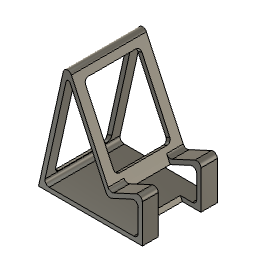
MultimeterStand (Autodesk Fusion 360 design; units mm, degrees)
Autodesk Fusion 360 part; units mm, degrees
sketch "Sketch11" plane through (0, 0, 0) normal (0, 1, 0) x (1, 0, 0)
  line L0 (0, 0) -> (0, -35) construction
  line L1 (0, -35) -> (38.0649, -52.75)
  line L2 (0, -35) -> (42, -35) construction
  line L3 (38.0649, -52.75) -> (38.0649, 0)
  line L4 (0, -35) -> (-48.0728, -138.0925)
  line L5 (0, -35) -> (131.25, -35) construction
  line L6 (-48.0728, -138.0925) -> (-53.0728, -138.0925)
  line L7 (0, 0) -> (61, 0) construction
  line L8 (-53.0728, -138.0925) -> (-83.6872, 0)
  line L9 (-53.0728, -138.0925) -> (72.8842, -138.0925) construction
  line L10 (0, 0) -> (-120, 0) construction
  line L11 (-83.6872, 0) -> (38.0649, 0)
  dimension "d68" = 35
  dimension "d69" = 42
  dimension "d70" = 25
  dimension "d71" = 115
  dimension "d72" = 113.75
  dimension "d73" = 5
  dimension "d81" = 102.5
  constraint vertical L0
  constraint coincident L0.start L7.start
  constraint horizontal L2
  constraint vertical L3
  constraint horizontal L5
  constraint horizontal L6
  constraint perpendicular L0 L7
  constraint coincident L3.end L7
  constraint horizontal L9
  constraint horizontal L10
  constraint coincident L8.end L10
  measures "d68" distance of L0.start L0.end
  measures "d69" distance of L0.end L1.end
  measures "d70" angle of L1 L2
  measures "d71" angle of L4 L5
  measures "d72" distance of L0.end L4.end
  measures "d73" distance of L4.end L6.end
  measures "d81" angle of L8 L9
extrude "Extrude16" add sketch "Sketch11" along normal blind 88
sketch "Sketch12" plane through (38.0649, 0, 0) normal (1, 0, 0) x (0, 1, 0)
  line L0 (0, 52.75) -> (0, 0)
  line L1 (88, 0) -> (88, 52.75)
  line L2 (88, 52.75) -> (0, 52.75)
  line L3 (44, 52.75) -> (43.2382, 0) construction
  line L4 (68.6191, 52.75) -> (18.6191, 52.75)
  line L5 (18.6191, 52.75) -> (18.6191, 0)
  line L6 (18.6191, 0) -> (68.6191, 0)
  line L7 (68.6191, 0) -> (68.6191, 52.75)
  line L8 (68.6191, 52.75) -> (18.6191, 0) construction
  line L9 (18.6191, 52.75) -> (68.6191, 0) construction
  line L10 (0, 0) -> (88, 0)
  point P0 (43.6191, 26.375)
  dimension "d77" = 50
  constraint midpoint L2 L3.start
  constraint horizontal L4
  constraint perpendicular L4 L5
  constraint parallel L4 L6
  constraint parallel L5 L7
  constraint coincident L8 P0
  constraint coincident L9 P0
  constraint midpoint L3 P0
  constraint coincident L3.end L10
  constraint collinear L2 L4
  measures "d77" distance of L5.end L6.end
extrude "Extrude17" cut sketch "Sketch12" along normal up to surface contours L2 L4 L5 L6 L7 L10 end surface through (0, 0, 35) normal (0.906308, 0, 0.422618) offset 0
sketch "Sketch13" plane through (0, 0, 0) normal (0, -1, 0) x (1, 0, 0)
  line L0 (38.0649, 52.75) -> (0, 35)
  line L1 (0, 35) -> (-48.0728, 138.0925)
  line L2 (-48.0728, 138.0925) -> (-53.0728, 138.0925)
  line L3 (-53.0728, 138.0925) -> (-83.6872, 0)
  line L4 (-83.6872, 0) -> (38.0649, 0)
  line L5 (38.0649, 0) -> (38.0649, 52.75)
  line L6 (33.0649, 5) -> (33.0649, 44.9015)
  line L7 (33.0649, 44.9015) -> (-2.4184, 28.3554)
  line L8 (-2.4184, 28.3554) -> (-49.7683, 129.8974)
  line L9 (-49.7683, 129.8974) -> (-77.4573, 5)
  line L10 (-77.4573, 5) -> (33.0649, 5)
extrude "Extrude18" cut sketch "Sketch13" against normal up to surface (88 mm away) contours L6 L7 L8 L9 L10
sketch "Sketch14" plane through (13.4058, 0, 6.2512) normal (0.906308, 0, 0.422618) x (0, 1, 0)
  line L0 (18.6191, 30.4685) -> (68.6191, 30.4685) construction
  line L1 (68.6191, 30.4685) -> (68.6191, 35) construction
  line L2 (68.6191, 35) -> (88, 35) construction
  line L3 (88, 35) -> (88, 138.0925) construction
  line L4 (88, 138.0925) -> (0, 138.0925) construction
  line L5 (0, 138.0925) -> (0, 35) construction
  line L6 (0, 35) -> (18.6191, 35) construction
  line L7 (18.6191, 35) -> (18.6191, 30.4685) construction
  line L8 (0, 138.0925) -> (88, 35) construction
  line L9 (72, 130.2963) -> (16, 130.2963)
  line L10 (11, 125.2963) -> (11, 47.7963)
  line L11 (16, 42.7963) -> (72, 42.7963)
  line L12 (77, 47.7963) -> (77, 125.2963)
  line L13 (77, 130.2963) -> (11, 42.7963) construction
  line L14 (11, 130.2963) -> (77, 42.7963) construction
  line L15 (18.6191, 26.7208) -> (68.6191, 26.7208)
  line L16 (68.6191, 26.7208) -> (68.6191, 31.7208)
  line L17 (68.6191, 31.7208) -> (88, 31.7208)
  line L18 (88, 31.7208) -> (88, 145.4708)
  line L19 (88, 145.4708) -> (0, 145.4708)
  line L20 (0, 145.4708) -> (0, 31.7208)
  line L21 (0, 31.7208) -> (18.6191, 31.7208)
  line L22 (18.6191, 31.7208) -> (18.6191, 26.7208)
  arc A0 (16, 130.2963) -> (11, 125.2963) centre (16, 125.2963) ccw
  arc A1 (77, 125.2963) -> (72, 130.2963) centre (72, 125.2963) ccw
  arc A2 (72, 42.7963) -> (77, 47.7963) centre (72, 47.7963) ccw
  arc A3 (11, 47.7963) -> (16, 42.7963) centre (16, 47.7963) ccw
  point P0 (44, 86.5463)
  dimension "d101" = 66
  dimension "d102" = 87.5
  dimension "d105" = 5
  constraint coincident L4.end L5.start
  constraint coincident L2.end L3.start
  constraint horizontal L9
  constraint perpendicular L9 L10
  constraint parallel L9 L11
  constraint parallel L10 L12
  constraint coincident L13 P0
  constraint coincident L14 P0
  constraint midpoint L8 P0
  constraint coincident L14.start L10
  constraint coincident L14.start L9
  constraint tangent L10 A0
  constraint tangent L9 A0
  constraint coincident L13.start L9
  constraint coincident L13.start L12
  constraint tangent L9 A1
  constraint tangent L12 A1
  constraint equal A0 A1
  constraint coincident L14.end L12
  constraint coincident L14.end L11
  constraint tangent L12 A2
  constraint tangent L11 A2
  constraint equal A0 A2
  constraint coincident L13.end L11
  constraint coincident L13.end L10
  constraint tangent L11 A3
  constraint tangent L10 A3
  constraint equal A0 A3
  measures "d101" distance of L13.end L14.end
  measures "d102" distance of L14.start L13.end
  measures "d105" radius of A0
fillet "Fillet5" radius 5 6 edges at (38.0649, 78.3095, 52.75) (38.0649, 9.3095, 52.75) (0, 9.3095, 35) (0, 78.3095, 35) (-48.0728, 44, 138.0925) (-53.0728, 44, 138.0925)
fillet "Fillet6" radius 2.5 1 edges at (-49.7683, 44, 129.8974)
fillet "Fillet6" radius 5 6 edges at (-77.4573, 44, 5) (33.0649, 9.3095, 5) (33.0649, 78.3095, 5) (33.0649, 78.3095, 44.9015) (33.0649, 9.3095, 44.9015) (-2.4184, 44, 28.3554)
extrude "Extrude19" cut sketch "Sketch14" along normal up to surface contours L9 L10 L11 L12 A0 A1 A2 A3 end surface through (-53.0728, 0, 138.0925) normal (-0.976296, 0, 0.21644) offset 0
equation "DeviceWidth = 88 mm"
equation "DeviceBottomThickness = 42 mm"
equation "Angle = 25 deg"
equation "DeviceHeight = 175 mm"
equation "WallThickness = 5 mm"
equation "ProbeDiameter = 9.7 mm"
equation "d69 = DeviceBottomThickness"
equation "d70 = Angle"
equation "d71 = Angle + 90 deg"
equation "d72 = DeviceHeight * 0.65"
equation "d73 = WallThickness"
equation "d74 = DeviceWidth"
equation "d81 = 90 deg + Angle / 2"
equation "d82 = -WallThickness"
equation "d86 = WallThickness"
equation "d96 = WallThickness"
equation "d100 = WallThickness / 2"
equation "d101 = DeviceWidth * 0.75"
equation "d102 = DeviceHeight * 0.5"
equation "d105 = WallThickness"
